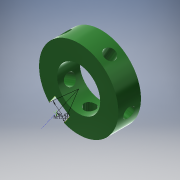
# Autodesk Inventor part: sprzeglo_04
Saved by Autodesk Inventor 2017 (Build 210142000, 142)
## iProperties
Created: 2021-05-22
Part Number: sprzeglo_04
Material: Generic
Document SubType Name: Modeling
Designer: majch
Density: 1 g/cm^3
Appearance: Smooth - Dark Forest Green
Mass: 5.60864 g
Surface Area: 35.0145 cm^2
Volume: 5.60864 cm^3
Author: majch
Autodesk Inventor part; units mm, degrees
sketch "Sketch1" plane through (0, 0, 0) normal (0, 1, 0) x (-1, 0, 0)
  circle A0 centre (0, 0) radius 17.5
  dimension "d0" = 35
  constraints: 1 centre point, 1 coincident
  measures "d0" diameter of A0
extrude "Extrusion1" add sketch "Sketch1" along normal blind 10
sketch "Sketch2" plane through (0, 10, 0) normal (0, 1, 0) x (1, 0, 0)
  circle A0 centre (0, 0) radius 9.5
  dimension "d3" = 19
  constraints: 1 centre point, 1 coincident
  measures "d3" diameter of A0
extrude "Extrusion2" cut sketch "Sketch2" against normal through all
ref_plane "Work Plane13" through (0, 0, 0) normal (0, 0, 1) x (0, 1, 0)
sketch "Sketch11" plane through (0, 0, 0) normal (0, 0, 1) x (0, 1, 0)
  circle A0 centre (5, 0) radius 2.5
  point P0 (0, 0)
  dimension "d52" = 5
  constraints: 1 centre point
  measures "d52" diameter of A0
hole "Hole5" at (0, 5, 0) direction (0, 0, -1) diameter 5 end through all
ref_plane "Work Plane14" through (0, 0, 0) normal (0.9397, 0, 0.342) x (0, 1, 0)
sketch "Sketch12" plane through (0, 0, 0) normal (0.9397, 0, 0.342) x (0, 1, 0)
  circle A0 centre (5, 0) radius 2.5
  point P0 (0, 0)
  dimension "d61" = 5
  constraints: 1 centre point
  measures "d61" diameter of A0
hole "Hole6" at (0, 5, 0) direction (-0.9397, 0, -0.342) diameter 5 end through all
ref_plane "Work Plane15" through (0, 0, 0) normal (0.6428, 0, -0.766) x (0, 1, 0)
sketch "Sketch13" plane through (0, 0, 0) normal (0.6428, 0, -0.766) x (0, 1, 0)
  circle A0 centre (5, 0) radius 2.5
  point P0 (0, 0)
  dimension "d70" = 5
  constraints: 1 centre point
  measures "d70" diameter of A0
hole "Hole7" at (0, 5, 0) direction (-0.6428, 0, 0.766) diameter 5 end through all
ref_plane "Work Plane16" through (0, 0, 0) normal (-0.5, 0, -0.866) x (0, 1, 0)
sketch "Sketch14" plane through (0, 0, 0) normal (-0.5, 0, -0.866) x (0, 1, 0)
  circle A0 centre (5, 0) radius 2.5
  point P0 (0, 0)
  dimension "d79" = 5
  constraints: 1 centre point
  measures "d79" diameter of A0
hole "Hole8" at (0, 5, 0) direction (0.5, 0, 0.866) diameter 5 end through all
ref_plane "Work Plane17" through (0, 0, 0) normal (-0.9848, 0, 0.1736) x (0, 1, 0)
sketch "Sketch15" plane through (0, 0, 0) normal (-0.9848, 0, 0.1736) x (0, 1, 0)
  circle A0 centre (5, 0) radius 2.5
  point P0 (0, 0)
  dimension "d88" = 5
  constraints: 1 centre point
  measures "d88" diameter of A0
hole "Hole9" at (0, 5, 0) direction (0.9848, 0, -0.1736) diameter 5 end through all
ref_plane "Work Plane21" through (-10.0376, 0, -14.3352) normal (0.5736, 0, 0.8192) x (0, 1, 0)
ref_plane "Work Plane20" through (0, 0, 0) normal (0.5736, 0, 0.8192) x (0, 1, 0)
sketch "Sketch16" plane through (-10.0376, 0, -14.3352) normal (0.5736, 0, 0.8192) x (0, 1, 0)
  line L0 (10, 4) -> (0, 4)
  line L1 (0, 4) -> (0, -4)
  line L2 (0, -4) -> (10, -4)
  line L3 (10, -4) -> (10, 4)
  line L4 (0, 17.5) -> (0, -17.5)
  line L5 (18.3389, 0) -> (-7, 0) construction
  point P0 (0, 0)
  dimension "d100" = 8
  dimension "d107" = 4
  dimension "d108" = 10
  constraints: 12 end point, 2 horizontal, 2 parallel, 1 perpendicular
  measures "d100" distance of L0.end L1.end
  measures "d107" distance between parallel lines of L5 L2
  measures "d108" distance of L0.start L0.end
extrude "Extrusion4" cut sketch "Sketch16" along normal blind 5
sketch "Sketch17" plane through (0, 0, 0) normal (0, -1, 0) x (1, 0, 0)
  line L0 (0, 0) -> (-16.3488, -23.3485) construction
  line L1 (-10.4463, -7.9451) -> (-13.0485, -11.6614) construction
  line L2 (-6.4953, -16.25) -> (-3.8931, -12.5337) construction
  line L3 (-3.8931, -12.5337) -> (-6.4953, -16.25) projected
  arc A0 (-6.4953, -16.25) -> (-13.0485, -11.6614) centre (0, 0) ccw projected
  line L4 (-13.0485, -11.6614) -> (-10.4463, -7.9451) projected
  line L5 (-10.4463, -7.9451) -> (-3.8931, -12.5337) projected
  circle A1 centre (0, 0) radius 9.5 projected
  point P0 (-10.0012, -14.2832)
  dimension "d114" = 26.426
  dimension "d115" = 13.213
  constraints: 2 end point, 1 point on line
equation "\"d107\" = 0.5 * d100"
equation "\"d115\" = 0.5 * d114"
body "Solid1"
